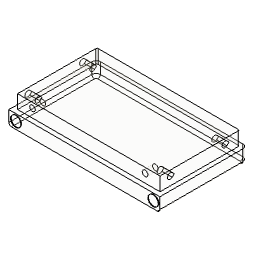
V3 U-shaped bottom + side panels v5 (Autodesk Fusion 360 archive; units mm, degrees)
design "V3 side panel"
Autodesk Fusion 360 part; units mm, degrees
sketch "base" plane through (0, 0, 0) normal (0, 0, 1) x (1, 0, 0)
  line L0 (0, 0) -> (88.5, 0)
  line L1 (88.5, 0) -> (88.5, 48.643)
  line L2 (86, 51.143) -> (2.5, 51.143)
  line L3 (0, 48.643) -> (0, 0)
  arc A0 (2.5, 51.143) -> (0, 48.643) centre (2.5, 48.643) ccw
  arc A1 (88.5, 48.643) -> (86, 51.143) centre (86, 48.643) ccw
  point P0 (0, 51.143)
  dimension "d1" = 88.5
  dimension "d2" = 51.143
  dimension "d14" = 2.5
  dimension "d15" = 2.5
  constraint horizontal L0
  constraint vertical L1
  constraint horizontal L2
  constraint vertical L3
  constraint coincident L0.start L3.end
  constraint coincident P0 L2
  constraint coincident P0 L3
  constraint tangent L2 A0
  constraint tangent L3 A0
  constraint tangent L1 A1
  constraint tangent L2 A1
  measures "d1" distance of L0.start L0.end
  measures "d2" distance of L0.start P0
  measures "d14" radius of A0
  measures "d15" radius of A1
extrude "Extrude1" add sketch "base" along normal blind 8
sketch "inside part" plane through (0, 0, 8) normal (0, 0, 1) x (-1, 0, 0)
  line L0 (0, -48.643) -> (0, 0)
  line L1 (0, 0) -> (-88.5, 0)
  line L2 (-88.5, 0) -> (-88.5, -48.643)
  line L3 (-86, -51.143) -> (-2.5, -51.143)
  line L4 (-2.5, 0) -> (-86, 0)
  line L5 (-86, 0) -> (-86, -48.381)
  line L6 (-85.238, -49.143) -> (-3.262, -49.143)
  line L7 (-2.5, -48.381) -> (-2.5, 0)
  arc A0 (-3.262, -49.143) -> (-2.5, -48.381) centre (-3.262, -48.381) ccw
  arc A1 (-86, -48.381) -> (-85.238, -49.143) centre (-85.238, -48.381) ccw
  arc A2 (-88.5, -48.643) -> (-86, -51.143) centre (-86, -48.643) ccw
  arc A3 (-2.5, -51.143) -> (0, -48.643) centre (-2.5, -48.643) ccw
  dimension "d7" = 2.5
  dimension "d8" = 2.5
  dimension "d9" = 2
  dimension "d12" = 0.762
  dimension "d13" = 0.762
  constraint horizontal L4
  constraint vertical L5
  constraint horizontal L6
  constraint vertical L7
  constraint coincident L1 L4.start
  constraint tangent L6 A0
  constraint tangent L7 A0
  constraint tangent L5 A1
  constraint tangent L6 A1
  measures "d7" distance of L0 L7
  measures "d8" distance of L2 L5
  measures "d9" distance of L3 L6
  measures "d12" radius of A0
  measures "d13" radius of A1
extrude "Extrude2" add sketch "inside part" along normal blind 8 contours L1 L4 L5 L6 L7 A0 A1
fillet "Fillet1" radius 1.5 5 edges at (88.5, 24.3215, 0) (87.7678, 50.4108, 0) (44.25, 51.143, 0) (0.7322, 50.4108, 0) (0, 24.3215, 0)
sketch "Sketch3" plane through (0, 0, 0) normal (0, -1, 0) x (1, 0, 0)
  arc A0 (87, 0) -> (88.5, 1.5) centre (87, 1.5) ccw
  line L0 (88.5, 1.5) -> (88.5, 8)
  line L1 (88.5, 8) -> (86, 8)
  line L2 (86, 8) -> (86, 16)
  line L3 (86, 16) -> (2.5, 16)
  line L4 (2.5, 16) -> (2.5, 8)
  line L5 (2.5, 8) -> (0, 8)
  line L6 (0, 8) -> (0, 1.5)
  arc A1 (0, 1.5) -> (1.5, 0) centre (1.5, 1.5) ccw
  line L7 (1.5, 0) -> (87, 0)
  line L8 (86, 8) -> (2.5, 8)
  line L9 (2.5, 8) -> (2.5, 16)
  line L10 (2.5, 16) -> (86, 16)
  line L11 (86, 16) -> (86, 8)
  constraint horizontal L8
  constraint vertical L9
  constraint horizontal L10
  constraint vertical L11
  constraint coincident L3.end L4.start
  constraint coincident L1.end L2.start
extrude "Extrude3" cut sketch "Sketch3" against normal blind 2.6 contours L2 L3 L4 L8 L9 L10 L11
sketch "Bottom holes for M2.5 screws" plane through (0, 2.6, 0) normal (0, -1, 0) x (1, 0, 0)
  line L0 (86, 16) -> (2.5, 16)
  line L1 (2.5, 16) -> (2.5, 8)
  line L2 (2.5, 8) -> (86, 8)
  line L3 (86, 8) -> (86, 16)
  line L4 (44.25, 8) -> (44.25, 16) construction
  point P0 (77.25, 13)
  point P1 (11.25, 13)
  dimension "d21" = 33
  dimension "d22" = 33
  dimension "d44" = 5
  constraint midpoint L2 L4.start
  constraint midpoint L0 L4.end
  constraint horizontal P0 P1
  measures "d21" distance of L4 P0
  measures "d22" distance of L4 P1
  measures "d44" distance of L2 P0
hole "Hole1" at (11.25, 2.6, 13) at (77.25, 2.6, 13) direction (0, 1, 0) diameter 3.3 depth 6 tip angle 180
sketch "Front/back holes" plane through (86, 0, 0) normal (1, 0, 0) x (0, 1, 0)
  line L0 (2.6, 16) -> (2.6, 8)
  line L1 (2.6, 8) -> (48.381, 8)
  line L2 (48.381, 8) -> (48.381, 16)
  line L3 (48.381, 16) -> (2.6, 16)
  circle A0 centre (8.6, 13) radius 1.65
  circle A1 centre (40.6, 13) radius 1.65
  line L4 (11, 13) -> (9.7344, 14.1982)
  line L5 (11, 13) -> (9.7344, 11.8018)
  line L6 (43, 13) -> (41.7344, 14.1982)
  line L7 (43, 13) -> (41.7344, 11.8018)
  point P0 (8.6, 13)
  point P1 (40.6, 13)
  dimension "d27" = 6
  dimension "d28" = 32
  dimension "d29" = 5
  dimension "d50" = 3.3
  dimension "d51" = 3.3
  dimension "d54" = 2.4
  dimension "d55" = 2.4
  constraint horizontal P0 P1
  constraint coincident P0 A0.centre
  constraint coincident P1 A1.centre
  constraint coincident A0 L4.end
  constraint tangent A0 L4
  constraint coincident A0 L5.end
  constraint tangent A0 L5
  constraint coincident A1 L6.end
  constraint tangent A1 L6
  constraint coincident A1 L7.end
  constraint tangent A1 L7
  constraint horizontal P0 L4.start
  constraint horizontal P1 L6.start
  measures "d27" distance of L0 P0
  measures "d28" distance of P0 P1
  measures "d29" distance of L1 P0
  measures "d50" diameter of A0
  measures "d51" diameter of A1
  measures "d54" distance of P0 L4.start
  measures "d55" distance of P1 L6.start
extrude "Extrude5" cut sketch "Front/back holes" against normal blind 6 contours A0 | A0 L4 L5 | A1 | A1 L6 L7
sketch "Front/back holes (1)" plane through (2.5, 0, 0) normal (-1, 0, 0) x (0, -1, 0)
  line L0 (-2.6, 8) -> (-2.6, 16)
  line L1 (-2.6, 16) -> (-48.381, 16)
  line L2 (-48.381, 16) -> (-48.381, 8)
  line L3 (-48.381, 8) -> (-2.6, 8)
  circle A0 centre (-40.6, 13) radius 1.65
  circle A1 centre (-8.6, 13) radius 1.65
  line L4 (-43, 13) -> (-41.7344, 11.8018)
  line L5 (-43, 13) -> (-41.7344, 14.1982)
  line L6 (-10.9921, 13) -> (-9.7381, 14.1947)
  line L7 (-10.9921, 13) -> (-9.7381, 11.8053)
  point P0 (-40.6, 13)
  point P1 (-8.6, 13)
  point P2 (-40.6, 13)
  point P3 (-40.6, 13)
  point P4 (-43, 13)
  point P5 (-8.6, 13)
  point P6 (-8.6, 13)
  point P7 (-11, 13)
  dimension "d33" = 6
  dimension "d34" = 32
  dimension "d45" = 5
  dimension "d46" = 3.3
  dimension "d47" = 3.3
  dimension "d56" = 2.4
  dimension "d57" = 2.4
  constraint horizontal P3 P1
  constraint coincident P3 P2
  constraint coincident P5 P1
  constraint coincident A0 L4.end
  constraint tangent A0 L4
  constraint coincident A0 L5.end
  constraint tangent A0 L5
  constraint coincident A1 L6.end
  constraint tangent A1 L6
  constraint coincident A1 L7.end
  constraint tangent A1 L7
  constraint horizontal L6.start P6
  constraint horizontal P3 P4
  measures "d33" distance of L0 P5
  measures "d34" distance of P3 P1
  measures "d45" distance of L3 P5
  measures "d46" diameter of A0
  measures "d47" diameter of A1
  measures "d56" distance of P3 P4
  measures "d57" distance of P6 P7
extrude "Extrude4" cut sketch "Front/back holes (1)" against normal blind 6 contours A0 | A0 L4 L5 | A1 | A1 L6 L7
sketch "Sketch8" plane through (0, 0, 0) normal (0, -1, 0) x (1, 0, 0)
  line L0 (88.5, 8) -> (0, 8)
  line L1 (0, 8) -> (0, 1.5)
  arc A0 (0, 1.5) -> (1.5, 0) centre (1.5, 1.5) ccw
  line L2 (1.5, 0) -> (87, 0)
  arc A1 (87, 0) -> (88.5, 1.5) centre (87, 1.5) ccw
  line L3 (88.5, 1.5) -> (88.5, 8)
  line L4 (88.5, 4) -> (0, 4) construction
  point P0 (4, 4)
  point P1 (84.5, 4)
  dimension "d58" = 4
  dimension "d59" = 4
  dimension "d60" = 4
  dimension "d61" = 4
  constraint coincident L3 L4.start
  constraint coincident L1 L4.end
  constraint perpendicular L1 L4
  constraint coincident L4 P0
  constraint coincident L4 P1
  measures "d58" distance of L0 L4
  measures "d59" distance of L0 L4.end
  measures "d60" distance of L4.end P0
  measures "d61" distance of L4.start P1
hole "Hole4" at (4, 0, 4) at (84.5, 0, 4) direction (0, 1, 0) diameter 6.1 depth 0.4 tip angle 180
equation "d1 = 83.5 mm + 2 * extrawidth"
equation "d2 = extraheight + 49.143 mm"
equation "extrawidth = 2.5 mm"
equation "extraheight = 2 mm"
equation "d7 = extrawidth"
equation "d8 = extrawidth"
equation "d9 = extraheight"
